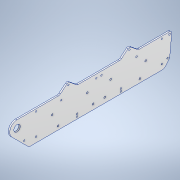
# Autodesk Inventor part: plyta_glowna_V3
Saved by Autodesk Inventor 2020.3 (Build 243373000, 373)
## iProperties
Created: 2021-04-10
Part Number: plyta_glowna_V3
Material: Aluminium 6061
Document SubType Name: Modeling
Designer: patryk.szydlik
Density: 2.7 g/cm^3
Appearance: Aluminium — płaski
Mass: 531.743 g
Surface Area: 1004.37 cm^2
Volume: 196.942 cm^3
Author: patryk.szydlik
Autodesk Inventor part; units mm, degrees
ref_plane "YZ Plane" through (0, 0, 0) normal (1, 0, 0) x (0, 1, 0)
ref_plane "XZ Plane" through (0, 0, 0) normal (0, 1, 0) x (-1, 0, 0)
ref_plane "XY Plane" through (0, 0, 0) normal (0, 0, 1) x (1, 0, 0)
sketch "Sketch2" plane through (0, 0, 0) normal (1, 0, 0) x (0, 1, 0)
  line L0 (127.2876, 96.9132) -> (-12.7124, 96.9132) construction
  line L1 (-12.7124, 96.9132) -> (-12.7124, -363.0868) construction
  line L2 (-12.7124, -363.0868) -> (127.2876, -363.0868) construction
  line L3 (127.2876, -363.0868) -> (127.2876, 96.9132) construction
  line L4 (97.2876, 66.9132) -> (17.2876, 66.9132) construction
  line L5 (17.2876, 66.9132) -> (17.2876, -333.0868) construction
  line L6 (17.2876, -333.0868) -> (97.2876, -333.0868) construction
  line L7 (97.2876, -333.0868) -> (97.2876, 66.9132) construction
  point P0 (0, 0)
  dimension "d2" = 140
  dimension "d3" = 460
  dimension "d4" = 80
  dimension "d5" = 400
  dimension "d6" = 30
  dimension "d7" = 30
  constraints: 16 end point, 4 parallel, 2 horizontal, 2 perpendicular
  measures "d2" distance of L2.end L1.end
  measures "d3" distance of L1.end L0.end
  measures "d4" distance of L6.end L5.end
  measures "d5" distance of L5.end L4.end
  measures "d6" distance between parallel lines of L3 L7
  measures "d7" distance between parallel lines of L0 L4
sketch "Sketch3" plane through (0, 0, 0) normal (1, 0, 0) x (0, 1, 0)
  circle A0 centre (-62.7124, 66.9132) radius 20
  line L0 (-12.7124, 96.9132) -> (-12.7124, -363.0868) construction
  circle A1 centre (-62.7124, -13.0868) radius 20
  circle A2 centre (-62.7124, -93.0868) radius 20
  circle A3 centre (-62.7124, -173.0868) radius 20
  circle A4 centre (-62.7124, -253.0868) radius 20
  circle A5 centre (-62.7124, -333.0868) radius 20
  line L1 (127.2876, 96.9132) -> (-12.7124, 96.9132) construction
  point P0 (0, 0)
  dimension "d8" = 40
  dimension "d9" = 50
  dimension "d12" = 80
  dimension "d17" = 30
  constraints: 6 centre point, 1 vertical, 10 other
  measures "d8" diameter of A0
  measures "d9" distance from line of L0 A0.centre
  measures "d12" distance of A0.centre A1.centre
  measures "d17" distance from line of A0.centre L1
sketch "Sketch1" plane through (0, 0, 0) normal (1, 0, 0) x (0, 1, 0)
  circle A0 centre (45.5719, 146.9132) radius 40
  circle A1 centre (85.5719, -453.0868) radius 40
  line L0 (127.2876, 96.9132) -> (-12.7124, 96.9132) construction
  line L1 (-12.7124, -363.0868) -> (127.2876, -363.0868) construction
  line L2 (-62.7124, 66.9132) -> (-62.7124, -13.0868) construction
  line L3 (-62.7124, -253.0868) -> (-62.7124, -333.0868) construction
  line L4 (85.2399, 141.7706) -> (125.4799, -450.3748) construction
  circle A2 centre (-62.7124, 66.9132) radius 20 projected
  line L5 (17.2876, 175.1975) -> (-76.8545, 81.0553)
  circle A3 centre (-62.7124, -333.0868) radius 20 projected
  line L6 (-76.8545, -347.2289) -> (57.2876, -481.3711) construction
  point P0 (0, 0)
  dimension "d0" = 80
  dimension "d1" = 80
  dimension "d18" = 50
  dimension "d19" = 90
  dimension "d45" = 135
  dimension "d46" = 135
  constraints: 10 end point, 4 point on circle, 3 tangent, 2 centre point, 2 coincident, 2 vertical, 6 other
  measures "d0" diameter of A0
  measures "d1" diameter of A1
  measures "d18" distance from line of A0.centre L0
  measures "d19" distance from line of A1.centre L1
  measures "d45" angle of L2 L5
  measures "d46" angle of L3 L6
sketch "Sketch4" plane through (0, 0, 0) normal (1, 0, 0) x (0, 1, 0)
  line L0 (37.6815, -3.0868) -> (-57.7124, 26.9132) construction
  circle A0 centre (-62.7124, 66.9132) radius 20 projected
  circle A1 centre (-62.7124, -13.0868) radius 20 projected
  line L1 (-62.7124, 66.9132) -> (-62.7124, -13.0868) construction
  circle A2 centre (-27.7124, 112.5679) radius 20 construction
  circle A3 centre (-27.7124, 32.5679) radius 20 construction
  line L2 (-27.7124, 72.5679) -> (37.6815, -3.0868) construction
  line L3 (-27.7124, 72.5679) -> (-57.7124, 26.9132) construction
  line L4 (37.6815, -3.0868) -> (-42.7124, 49.7406) construction
  line L5 (-12.7124, 96.9132) -> (-12.7124, -363.0868) construction
  point P0 (0, 0)
  point P1 (-61.7124, 47.9132)
  point P2 (83.0715, 79.9132)
  point P3 (83.0715, -80.0868)
  point P4 (37.6815, -163.0868)
  point P5 (83.0715, -240.0868)
  point P6 (37.6815, -323.0868)
  dimension "d22" = 40
  dimension "d23" = 5
  dimension "d24" = 30
  dimension "d25" = 40
  dimension "d26" = 40
  dimension "d27" = 80
  dimension "d28" = 40
  dimension "d29" = 100
  dimension "d30" = 100
  dimension "d31" = 35
  dimension "d32" = 54.6292
  dimension "d33" = 27.3146
  dimension "d34" = 56.691
  dimension "d35" = 95.3939
  dimension "d36" = 45.39
  dimension "d37" = 83
  dimension "d40" = 160
  constraints: 8 end point, 2 centre point, 2 vertical alignment, 1 coincident, 1 midpoint, 1 vertical, 4 other
  measures "d22" vertical distance of point (-62.712, 66.913) L0.end
  measures "d23" horizontal distance of point (-62.712, 66.913) L0.end
  measures "d24" vertical distance of L0.end L0.start
  measures "d25" diameter of A3
  measures "d26" diameter of A2
  measures "d27" distance of A3.centre A2.centre
  measures "d28" distance of A3.centre L2.start
  measures "d29" distance of L0.start L0.end
  measures "d30" distance of L2.start L0.start
  measures "d31" horizontal distance of point (-62.712, 66.913) A2.centre
  measures "d32" distance of L0.end L2.start
  measures "d33" distance of L0.end L4.end
  measures "d34" angle of L5 L4
  measures "d35" horizontal distance of L0.end L0.start
  measures "d36" horizontal distance of L0.start point (83.072, 79.913)
  measures "d37" vertical distance of L0.start point (83.072, 79.913)
  measures "d40" distance of point (83.072, 79.913) point (83.072, -80.087)
sketch "Sketch6" plane through (0, 0, 0) normal (1, 0, 0) x (0, 1, 0)
  line L0 (234.6261, -208.0868) -> (-157.479, -208.0868) construction
  line L1 (237.7494, -58.0868) -> (-154.3557, -58.0868) construction
  line L2 (17.2876, -333.0868) -> (97.2876, -333.0868) construction
  line L3 (97.2876, 66.9132) -> (17.2876, 66.9132) construction
  point P0 (0, 0)
  dimension "d61" = 125
  dimension "d62" = 125
  constraints: 4 end point, 2 horizontal
  measures "d61" distance between parallel lines of L1 L3
  measures "d62" distance between parallel lines of L2 L0
sketch "Sketch5" plane through (0, 0, 0) normal (1, 0, 0) x (0, 1, 0)
  arc A0 (90.5716, 146.9132) -> (47.894, 164.5909) centre (65.5716, 146.9132) ccw
  arc A1 (47.894, 164.5909) -> (90.5716, 146.9132) centre (65.5716, 146.9132) ccw construction
  line L0 (110.6559, 96.9132) -> (-29.3441, 96.9132) construction
  line L1 (-26.0812, -363.0868) -> (113.9188, -363.0868) construction
  line L2 (217.7491, -58.0868) -> (-174.356, -58.0868) construction
  line L3 (214.6258, -208.0868) -> (-177.4793, -208.0868) construction
  circle A2 centre (65.5716, 146.9132) radius 11
  circle A3 centre (65.5716, 146.9132) radius 55 construction
  line L4 (-10.2747, 106.4223) -> (47.894, 164.5909)
  line L5 (12.4387, 66.0715) -> (12.4387, -333.9285) construction
  line L6 (-62.7124, -14.3648) -> (-62.7124, -91.8088) construction
  line L7 (-62.7124, -173.0868) -> (-62.7124, -253.0868) construction
  line L8 (90.5716, -363.0868) -> (90.5716, -271.0908)
  line L9 (90.5716, -363.0868) -> (90.5716, -374.7257)
  arc A4 (82.3188, -382.1878) -> (90.5716, -374.7257) centre (83.0716, -374.7257) ccw
  arc A5 (11.0193, -373.8083) -> (14.9188, -375.3878) centre (15.6716, -367.9257) ccw
  line L10 (82.3188, -382.1878) -> (14.9188, -375.3878)
  arc A6 (-10.2747, -348.0868) -> (-3.3089, -362.4767) centre (8.0716, -348.0868) ccw
  line L11 (11.0193, -373.8083) -> (-3.3089, -362.4767)
  line L12 (-10.2747, -348.0868) -> (-10.2747, 106.4223)
  circle A7 centre (105.5716, -28.6718) radius 15 construction
  circle A8 centre (105.5716, -237.5018) radius 15 construction
  arc A9 (111.36, -33.441) -> (111.36, -23.9026) centre (105.5716, -28.6718) ccw
  arc A10 (111.36, -242.271) -> (111.36, -232.7326) centre (105.5716, -237.5018) ccw
  line L13 (111.36, -232.7326) -> (92.8538, -210.2717)
  line L14 (111.36, -242.271) -> (92.8538, -264.7319)
  line L15 (111.36, -33.441) -> (92.8538, -55.9019)
  line L16 (111.36, -23.9026) -> (92.8538, -1.4417)
  line L17 (90.5716, 4.9172) -> (90.5716, 146.9132)
  arc A11 (90.5716, 4.9172) -> (92.8538, -1.4417) centre (100.5716, 4.9172) ccw
  arc A12 (92.8538, -55.9019) -> (90.5716, -62.2608) centre (100.5716, -62.2608) ccw
  line L18 (90.5716, -203.9128) -> (90.5716, -62.2608)
  arc A13 (90.5716, -203.9128) -> (92.8538, -210.2717) centre (100.5716, -203.9128) ccw
  arc A14 (92.8538, -264.7319) -> (90.5716, -271.0908) centre (100.5716, -271.0908) ccw
  line L19 (127.2876, -363.0868) -> (127.2876, 96.9132) construction
  point P0 (0, 0)
  point P1 (83.0716, 81.9132)
  point P2 (83.0716, -348.0868)
  point P3 (16.3276, 122.4179)
  point P4 (8.0716, -82.4742)
  point P5 (8.0716, -243.0868)
  point P6 (-2.5613, -58.0868)
  point P7 (-2.5613, -208.0868)
  point P8 (8.0716, 81.9132)
  point P9 (-62.7124, 66.9132)
  point P10 (-62.7124, -333.0868)
  point P11 (-62.7124, -53.0868)
  point P12 (-62.7124, -213.0868)
  point P13 (2.2876, 6.9132)
  point P14 (45.3216, 26.9132)
  point P15 (50.3216, -93.0868)
  point P16 (7.2876, -113.0868)
  point P17 (7.2876, -153.0868)
  point P18 (50.3216, -173.0868)
  point P19 (45.3216, -293.0868)
  point P20 (2.2876, -273.0868)
  point P21 (2.2876, 6.9132)
  point P22 (-62.7124, 66.9132)
  point P23 (5.5716, -208.0868)
  point P24 (5.5716, -58.0868)
  point P25 (73.0216, -4.2568)
  point P26 (78.0216, -124.2568)
  point P27 (78.0216, -141.9168)
  point P28 (73.0216, -261.9168)
  point P29 (90.5716, -207.5018)
  point P30 (90.5716, -267.5018)
  point P31 (90.5716, -58.6718)
  point P32 (90.5716, 1.3282)
  point P33 (90.5716, -58.0868)
  point P34 (15.0521, -366.9249)
  dimension "d84" = 110
  dimension "d47" = 50
  dimension "d63" = 15
  dimension "d65" = 15
  dimension "d81" = 22
  dimension "d101" = 7.5
  dimension "d151" = 15
  dimension "d155" = 15
  dimension "d159" = 15
  dimension "d163" = 60
  dimension "d164" = 65
  dimension "d165" = 20
  dimension "d166" = 43.034
  dimension "d174" = 60
  dimension "d175" = 70
  dimension "d176" = 43.034
  dimension "d177" = 20
  dimension "d196" = 128.284
  dimension "d198" = 11.17
  dimension "d199" = 70.734
  dimension "d200" = 11.17
  dimension "d201" = 70.734
  dimension "d204" = 11.17
  dimension "d214" = 43.034
  dimension "d215" = 20
  dimension "d216" = 20
  dimension "d217" = 43.034
  dimension "d218" = 70.734
  dimension "d219" = 70.734
  dimension "d220" = 11.17
  dimension "d221" = 67.4
  dimension "d222" = 6.8
  dimension "d223" = 7.5
  dimension "d224" = 15
  dimension "d225" = 15
  dimension "d226" = 48.83
  dimension "d227" = 24.415
  dimension "d228" = 48.83
  dimension "d229" = 24.415
  dimension "d230" = 15
  dimension "d231" = 15
  dimension "d232" = 30
  dimension "d233" = 30
  dimension "d234" = 15
  dimension "d235" = 15
  dimension "d236" = 60
  dimension "d237" = 30
  dimension "d238" = 60
  dimension "d239" = 30
  dimension "d240" = 10
  dimension "d241" = 10
  dimension "d243" = 65
  dimension "d244" = 17.5
  dimension "d245" = 75
  dimension "d246" = 164.3874
  constraints: 38 end point, 22 point on circle, 17 tangent, 16 point on line, 14 centre point, 13 vertical alignment, 11 coincident, 2 equal radius, 2 midpoint, 2 vertical, 1 horizontal, 1 horizontal alignment, 8 other
  measures "d47" diameter of A0
  measures "d63" distance from line of L0 point (83.072, 81.913)
  measures "d65" distance from line of L1 point (83.072, -348.087)
  measures "d81" diameter of A2
  measures "d101" distance from line of point (16.328, 122.418) L4
  measures "d151" distance from line of L5 point (-2.561, -58.087)
  measures "d155" distance from line of L5 point (-2.561, -208.087)
  measures "d159" distance from line of L0 point (8.072, 81.913)
  measures "d163" vertical distance of point (-62.712, 66.913) point (2.288, 6.913)
  measures "d164" horizontal distance of point (-62.712, 66.913) point (2.288, 6.913)
  measures "d165" vertical distance of point (2.288, 6.913) point (45.322, 26.913)
  measures "d166" horizontal distance of point (2.288, 6.913) point (45.322, 26.913)
  measures "d174" vertical distance of point (-62.712, -213.087) point (7.288, -153.087)
  measures "d175" horizontal distance of point (-62.712, -213.087) point (7.288, -153.087)
  measures "d176" horizontal distance of point (50.322, -173.087) point (7.288, -153.087)
  measures "d177" vertical distance of point (50.322, -173.087) point (7.288, -153.087)
  measures "d196" horizontal distance of point (65.572, 146.913) point (-62.712, 66.913)
  measures "d198" vertical distance of point (73.022, -4.257) point (2.288, 6.913)
  measures "d199" horizontal distance of point (2.288, 6.913) point (73.022, -4.257)
  measures "d200" vertical distance of point (7.288, -113.087) point (78.022, -124.257)
  measures "d201" horizontal distance of point (7.288, -113.087) point (78.022, -124.257)
  measures "d204" vertical distance of point (2.288, -273.087) point (73.022, -261.917)
  measures "d214" horizontal distance of point (2.288, -273.087) point (45.322, -293.087)
  measures "d215" vertical distance of point (2.288, -273.087) point (45.322, -293.087)
  measures "d216" vertical distance of point (7.288, -113.087) point (50.322, -93.087)
  measures "d217" horizontal distance of point (50.322, -93.087) point (7.288, -113.087)
  measures "d218" horizontal distance of point (7.288, -153.087) point (78.022, -141.917)
  measures "d219" horizontal distance of point (2.288, -273.087) point (73.022, -261.917)
  measures "d220" vertical distance of point (7.288, -153.087) point (78.022, -141.917)
  measures "d221" horizontal distance of point (15.672, -367.926) point (83.072, -374.726)
  measures "d222" vertical distance of point (15.672, -367.926) point (83.072, -374.726)
  measures "d223" distance from line of L8 point (83.072, -374.726)
  measures "d224" diameter of A4
  measures "d225" diameter of A5
  measures "d226" vertical distance of point (-62.712, -53.087) point (73.022, -4.257)
  measures "d227" vertical distance of point (73.022, -4.257) point (105.572, -28.672)
  measures "d228" vertical distance of point (-62.712, -213.087) point (73.022, -261.917)
  measures "d229" vertical distance of point (73.022, -261.917) point (105.572, -237.502)
  measures "d230" distance from line of L8 point (105.572, -28.672)
  measures "d231" distance from line of L8 point (105.572, -237.502)
  measures "d232" diameter of A7
  measures "d233" diameter of A8
  measures "d234" diameter of A9
  measures "d235" diameter of A10
  measures "d236" distance of point (90.572, -58.672) point (90.572, 1.328)
  measures "d237" vertical distance of point (90.572, 1.328) point (105.572, -28.672)
  measures "d238" distance of point (90.572, -267.502) point (90.572, -207.502)
  measures "d239" vertical distance of A8.centre point (90.572, -207.502)
  measures "d240" radius of A11
  measures "d241" radius of A13
  measures "d243" vertical distance of point (65.572, 146.913) point (83.072, 81.913)
  measures "d244" horizontal distance of point (83.072, 81.913) point (65.572, 146.913)
  measures "d245" distance of point (83.072, 81.913) point (8.072, 81.913)
  measures "d246" distance of point (8.072, -82.474) point (8.072, 81.913)
extrude "Extrusion1" add sketch "Sketch5" against normal blind 5
hole "Hole1" at (0, 83.0716, 81.9132) at (0, 16.3276, 122.4179) at (0, 8.0716, -348.0868) at (0, 83.0716, -348.0868) at (0, -2.5613, -58.0868) at (0, -2.5613, -208.0868) at (0, 8.0716, 81.9132) at (0, 5.5716, -58.0868) at (0, 5.5716, -208.0868) at (0, 105.5716, -28.6718) at (0, 105.5716, -237.5018) direction (-1, 0, 0) diameter 5 end through all clearance for "Flat Head Machine Screw" size "M5" standard "Ansi Metric M Profile"
hole "Otwór2" at (0, 2.2876, 6.9132) at (0, 45.3216, 26.9132) at (0, 7.2876, -113.0868) at (0, 50.3216, -93.0868) at (0, 7.2876, -153.0868) at (0, 50.3216, -173.0868) at (0, 2.2876, -273.0868) at (0, 45.3216, -293.0868) at (0, 83.0716, -374.7257) direction (-1, 0, 0) diameter 6 end through all
hole "Otwór3" at (0, 73.0216, -4.2568) at (0, 78.0216, -141.9168) at (0, 78.0216, -124.2568) at (0, 73.0216, -261.9168) at (0, 15.6716, -367.9257) direction (-1, 0, 0) diameter 5 end through all
equation "\"d28\" = 0.5 * d27"
equation "\"d30\" = d29"
equation "\"d33\" = 0.5 * d32"
equation "\"d62\" = d61"
body "Solid1"
